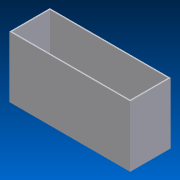
# Autodesk Inventor part: Small Battery Box Pastic 1
Saved by Autodesk Inventor 2012 (Build 160160000, 160)
## iProperties
Created: 2012-07-01
Part Number: Small Battery Box Pastic 1
Material: Default
Document SubType Name: Modeling
Designer: Hemant
Density: 1 g/cm^3
Author: Hemant
Autodesk Inventor part; units mm, degrees
ref_plane "YZ Plane" through (0, 0, 0) normal (1, 0, 0) x (0, 1, 0)
ref_plane "XZ Plane" through (0, 0, 0) normal (0, 1, 0) x (-1, 0, 0)
ref_plane "XY Plane" through (0, 0, 0) normal (0, 0, 1) x (1, 0, 0)
sketch "Sketch1" plane through (0, 0, 0) normal (0, 0, 1) x (1, 0, 0)
  line L0 (0, 0) -> (558.8, 0)
  line L1 (558.8, 0) -> (558.8, 282.575)
  line L2 (558.8, 282.575) -> (0, 282.575)
  line L3 (0, 282.575) -> (0, 0)
  dimension "d0" = 558.8
  dimension "d1" = 282.575
  constraints: 8 end point, 2 parallel, 1 horizontal, 1 perpendicular
  measures "d0" distance between parallel lines of L1 L3
  measures "d1" distance between parallel lines of L2 L0
extrude "Extrusion1" add sketch "Sketch1" along normal blind 187.325
sketch "Sketch2" plane through (0, 282.575, 0) normal (0, 1, 0) x (1, 0, 0)
  line L0 (0, -187.325) -> (558.8, -187.325) projected
  line L1 (0, 0) -> (0, -187.325) projected
  line L2 (6.35, -180.975) -> (552.45, -180.975)
  line L3 (552.45, -180.975) -> (552.45, -6.35)
  line L4 (552.45, -6.35) -> (6.35, -6.35)
  line L5 (6.35, -6.35) -> (6.35, -180.975)
  dimension "d4" = 6.35
  dimension "d5" = 6.35
  dimension "d6" = 546.1
  dimension "d7" = 174.625
  constraints: 8 end point, 2 parallel, 1 horizontal, 1 perpendicular
  measures "d4" distance between parallel lines of L5 L1
  measures "d5" distance between parallel lines of L0 L2
  measures "d6" distance between parallel lines of L3 L5
  measures "d7" distance between parallel lines of L4 L2
extrude "Extrusion2" cut sketch "Sketch2" against normal blind 276.225
body "Solid1"
